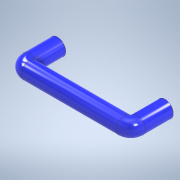
# Autodesk Inventor part: mango_zona_calor
Saved by Autodesk Inventor 2021 (Build 250183000, 183)
## iProperties
Created: 2021-04-15
Part Number: mango_zona_calor
Material: Plástico PC/ABS
Document SubType Name: Modeling
Designer: Leonardo Fabio Mercado Benítez
Density: 0.357273 g/cm^3
Appearance: Suave - Blanco
Mass: 22.9351 g
Surface Area: 141.565 cm^2
Volume: 64.195 cm^3
Author: Leonardo Fabio Mercado Benítez
Autodesk Inventor part; units mm, degrees
ref_plane "YZ Plane" through (0, 0, 0) normal (1, 0, 0) x (0, 1, 0)
ref_plane "XZ Plane" through (0, 0, 0) normal (0, 1, 0) x (-1, 0, 0)
ref_plane "XY Plane" through (0, 0, 0) normal (0, 0, 1) x (1, 0, 0)
sketch "Boceto1" plane through (0, 0, 0) normal (0, 1, 0) x (-1, 0, 0)
  line L0 (0, 0) -> (65, 0) construction
  line L1 (0, 0) -> (-65, 0) construction
  line L2 (65, 0) -> (65, 34)
  line L3 (-65, 0) -> (-65, 34)
  line L4 (65, 34) -> (57.5, 34) construction
  line L5 (-65, 34) -> (-57.5, 34) construction
  arc A0 (65, 34) -> (57.5, 41.5) centre (57.5, 34) ccw
  arc A1 (-57.5, 41.5) -> (-65, 34) centre (-57.5, 34) ccw
  line L6 (-57.5, 41.5) -> (57.5, 41.5)
  dimension "d0" = 65
  dimension "d1" = 65
  dimension "d2" = 34
  dimension "d3" = 34
  dimension "d5" = 7.5
  dimension "d6" = 7.5
  constraints: 14 end point, 5 horizontal, 4 point on circle, 2 centre point, 2 coincident, 2 vertical
  measures "d0" distance of L0.start L0.end
  measures "d1" distance of L0.start L1.end
  measures "d2" distance of L0.end L2.end
  measures "d3" distance of L1.end L3.end
  measures "d5" distance of L2.end L4.end
  measures "d6" distance of L3.end L5.end
sketch "Boceto2" plane through (0, 0, 0) normal (0, 0, 1) x (1, 0, 0)
  circle A0 centre (-65, 0) radius 10
  point P0 (0, 0)
  dimension "d7" = 20
  constraints: 1 centre point
  measures "d7" diameter of A0
sweep "Barrido1" add profiles "Boceto2" path "Boceto1"
sketch "Boceto3" plane through (65, 0, 0) normal (0, 0, -1) x (-1, 0, 0)
  circle A0 centre (0, 0) radius 2.3813
  circle A1 centre (130, 0) radius 2.3812
  point P0 (65, 0)
  dimension "d10" = 4.7625
  dimension "d11" = 4.7625
  constraints: 3 coincident, 2 centre point
  measures "d10" diameter of A0
  measures "d11" diameter of A1
extrude "Extrusión1" cut sketch "Boceto3" against normal blind 19.05
